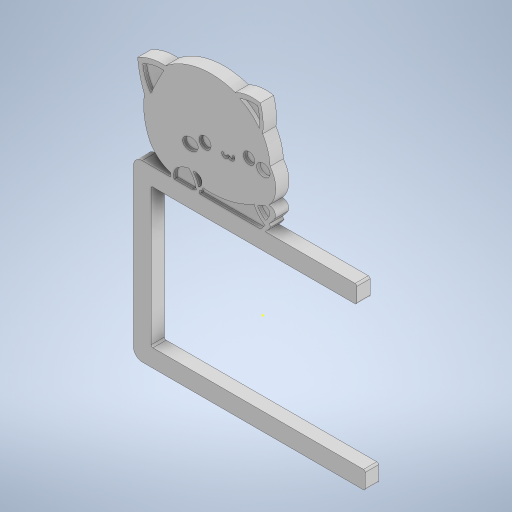
# Autodesk Inventor part: Top_Left
Saved by Autodesk Inventor 2023 (Build 270158000, 158)
## iProperties
Created: 2022-11-13
Part Number: Top_Left
Material: Generic
Document SubType Name: Modeling
Designer: reide
Density: 1 g/cm^3
Appearance: Default
Author: reide
Autodesk Inventor part; units mm, degrees
ref_plane "YZ Plane" through (0, 0, 0) normal (1, 0, 0) x (0, 1, 0)
ref_plane "XZ Plane" through (0, 0, 0) normal (0, 1, 0) x (-1, 0, 0)
ref_plane "XY Plane" through (0, 0, 0) normal (0, 0, 1) x (1, 0, 0)
sketch "Sketch1" plane through (0, 0, 0) normal (0, 0, 1) x (1, 0, 0)
  line L0 (44.2692, 42.6) -> (44.2692, 40.35) projected
  arc A0 (44.2692, 40.35) -> (45.2692, 39.35) centre (45.2692, 40.35) ccw projected
  line L1 (45.2692, 39.35) -> (59.7692, 39.35) projected
  arc A1 (59.7692, 39.35) -> (60.7692, 40.35) centre (59.7692, 40.35) ccw projected
  line L2 (60.7692, 40.35) -> (60.7692, 48.35) projected
  arc A2 (60.7692, 48.35) -> (59.7692, 49.35) centre (59.7692, 48.35) ccw projected
  line L3 (59.7692, 49.35) -> (-60.5312, 49.35) projected
  arc A3 (-60.5312, 49.35) -> (-65.5312, 44.35) centre (-60.5312, 44.35) ccw projected
  line L4 (-65.5312, 44.35) -> (-65.5312, -44.35) projected
  arc A4 (-65.5312, -44.35) -> (-60.5312, -49.35) centre (-60.5312, -44.35) ccw projected
  line L5 (-60.5312, -49.35) -> (64.5312, -49.35) projected
  arc A5 (64.5312, -49.35) -> (65.5312, -48.35) centre (64.5312, -48.35) ccw projected
  line L6 (65.5312, -48.35) -> (65.5312, -40.35) projected
  arc A6 (65.5312, -40.35) -> (64.5312, -39.35) centre (64.5312, -40.35) ccw projected
  line L7 (64.5312, -39.35) -> (49.5062, -39.35) projected
  line L8 (49.5062, -39.35) -> (49.5062, -41.65) projected
  arc A7 (48.5062, -42.65) -> (49.5062, -41.65) centre (48.5062, -41.65) ccw projected
  line L9 (48.5062, -42.65) -> (29.9062, -42.65) projected
  arc A8 (28.9062, -41.65) -> (29.9062, -42.65) centre (29.9062, -41.65) ccw projected
  line L10 (28.9062, -41.65) -> (28.9062, -39.35) projected
  line L11 (28.9062, -39.35) -> (-18.4058, -39.35) projected
  line L12 (-18.4058, -39.35) -> (-18.4058, -41.65) projected
  arc A9 (-19.4058, -42.65) -> (-18.4058, -41.65) centre (-19.4058, -41.65) ccw projected
  line L13 (-19.4058, -42.65) -> (-38.0058, -42.65) projected
  arc A10 (-39.0058, -41.65) -> (-38.0058, -42.65) centre (-38.0058, -41.65) ccw projected
  line L14 (-39.0058, -41.65) -> (-39.0058, -39.35) projected
  line L15 (-39.0058, -39.35) -> (-54.5312, -39.35) projected
  arc A11 (-55.5312, -38.35) -> (-54.5312, -39.35) centre (-54.5312, -38.35) ccw projected
  line L16 (-55.5312, -38.35) -> (-55.5312, -17.1) projected
  arc A12 (-55.5312, -17.1) -> (-56.5312, -16.1) centre (-56.5312, -17.1) ccw projected
  line L17 (-56.5312, -16.1) -> (-58.7812, -16.1) projected
  arc A13 (-59.7812, -15.1) -> (-58.7812, -16.1) centre (-58.7812, -15.1) ccw projected
  line L18 (-59.7812, -15.1) -> (-59.7812, -4.1) projected
  arc A14 (-58.7812, -3.1) -> (-59.7812, -4.1) centre (-58.7812, -4.1) ccw projected
  line L19 (-58.7812, -3.1) -> (-56.5312, -3.1) projected
  arc A15 (-56.5312, -3.1) -> (-55.5312, -2.1) centre (-56.5312, -2.1) ccw projected
  line L20 (-55.5312, -2.1) -> (-55.5312, 2.225) projected
  line L21 (-55.5312, 2.225) -> (-57.8308, 2.225) projected
  arc A16 (-58.8308, 3.225) -> (-57.8308, 2.225) centre (-57.8308, 3.225) ccw projected
  line L22 (-58.8308, 3.225) -> (-58.8308, 21.825) projected
  arc A17 (-57.8308, 22.825) -> (-58.8308, 21.825) centre (-57.8308, 21.825) ccw projected
  line L23 (-57.8308, 22.825) -> (-55.5312, 22.825) projected
  line L24 (-55.5312, 22.825) -> (-55.5312, 38.35) projected
  arc A18 (-54.5312, 39.35) -> (-55.5312, 38.35) centre (-54.5312, 38.35) ccw projected
  line L25 (-54.5312, 39.35) -> (-39.0058, 39.35) projected
  line L26 (-39.0058, 39.35) -> (-39.0058, 41.65) projected
  arc A19 (-38.0058, 42.65) -> (-39.0058, 41.65) centre (-38.0058, 41.65) ccw projected
  line L27 (-38.0058, 42.65) -> (-19.4058, 42.65) projected
  arc A20 (-18.4058, 41.65) -> (-19.4058, 42.65) centre (-19.4058, 41.65) ccw projected
  line L28 (-18.4058, 41.65) -> (-18.4058, 39.35) projected
  line L29 (-18.4058, 39.35) -> (0.3317, 39.35) projected
  line L30 (0.3317, 39.35) -> (0.3317, 41.65) projected
  arc A21 (1.3317, 42.65) -> (0.3317, 41.65) centre (1.3317, 41.65) ccw projected
  line L31 (1.3317, 42.65) -> (19.9317, 42.65) projected
  arc A22 (20.9317, 41.65) -> (19.9317, 42.65) centre (19.9317, 41.65) ccw projected
  line L32 (20.9317, 41.65) -> (20.9317, 39.35) projected
  line L33 (20.9317, 39.35) -> (25.2692, 39.35) projected
  arc A23 (25.2692, 39.35) -> (26.2692, 40.35) centre (25.2692, 40.35) ccw projected
  line L34 (26.2692, 40.35) -> (26.2692, 42.35) projected
  arc A24 (25.2692, 41.35) -> (26.2692, 42.35) centre (25.2692, 42.35) ccw projected
  line L35 (25.2692, 41.35) -> (21.9317, 41.35) projected
  arc A25 (20.9317, 42.35) -> (21.9317, 41.35) centre (21.9317, 42.35) ccw projected
  line L36 (20.9317, 44.2959) -> (20.9317, 42.35) projected
  ellipse E0 centre (21.9317, 44.2959) end of major axis (21.9317, 43.2418) minor radius 1 (21.9317, 45.35) -> (20.9317, 44.2959) ccw projected
  line L37 (21.9317, 45.35) -> (34.9317, 45.35) projected
  ellipse E1 centre (34.9317, 44.2959) end of major axis (34.9317, 43.2418) minor radius 1 (35.9207, 44.452) -> (34.9317, 45.35) ccw projected
  arc A26 (34.9317, 43.6) -> (35.9207, 44.452) centre (34.9317, 44.6) ccw projected
  line L38 (34.9317, 43.6) -> (43.2692, 43.6) projected
  arc A27 (44.2692, 42.6) -> (43.2692, 43.6) centre (43.2692, 42.6) ccw projected
  arc A28 (-39.0058, -42.35) -> (-40.0058, -41.35) centre (-40.0058, -42.35) ccw projected
  line L39 (-39.0058, -44.2959) -> (-39.0058, -42.35) projected
  ellipse E2 centre (-40.0058, -44.2959) end of major axis (-40.0058, -43.2418) minor radius 1 (-40.0058, -45.35) -> (-39.0058, -44.2959) ccw projected
  line L40 (-40.0058, -45.35) -> (-53.0057, -45.35) projected
  ellipse E3 centre (-53.0057, -44.2959) end of major axis (-53.0057, -43.2418) minor radius 1 (-54.0057, -44.2959) -> (-53.0057, -45.35) ccw projected
  line L41 (-54.0057, -42.35) -> (-54.0057, -44.2959) projected
  arc A29 (-53.0057, -41.35) -> (-54.0057, -42.35) centre (-53.0057, -42.35) ccw projected
  line L42 (-53.0057, -41.35) -> (-40.0058, -41.35) projected
  circle A30 centre (55.7692, 44.35) radius 2.125 projected
  circle A31 centre (-60.5312, 44.35) radius 2.125 projected
  circle A32 centre (-60.5312, -44.35) radius 2.125 projected
  circle A33 centre (60.5312, -44.35) radius 2.125 projected
  line L43 (-40.0058, 41.35) -> (-53.0058, 41.35) projected
  arc A34 (-54.0058, 42.35) -> (-53.0058, 41.35) centre (-53.0058, 42.35) ccw projected
  line L44 (-54.0058, 44.2959) -> (-54.0058, 42.35) projected
  ellipse E4 centre (-53.0058, 44.2959) end of major axis (-53.0058, 43.2418) minor radius 1 (-53.0058, 45.35) -> (-54.0058, 44.2959) ccw projected
  line L45 (-53.0058, 45.35) -> (-40.0058, 45.35) projected
  ellipse E5 centre (-40.0058, 44.2959) end of major axis (-40.0058, 43.2418) minor radius 1 (-39.0058, 44.2959) -> (-40.0058, 45.35) ccw projected
  line L46 (-39.0058, 42.35) -> (-39.0058, 44.2959) projected
  arc A35 (-40.0058, 41.35) -> (-39.0058, 42.35) centre (-40.0058, 42.35) ccw projected
  arc A36 (28.9062, -42.35) -> (27.9062, -41.35) centre (27.9062, -42.35) ccw projected
  line L47 (28.9062, -44.2959) -> (28.9062, -42.35) projected
  ellipse E6 centre (27.9062, -44.2959) end of major axis (27.9062, -43.2418) minor radius 1 (27.9063, -45.35) -> (28.9062, -44.2959) ccw projected
  line L48 (27.9063, -45.35) -> (14.9063, -45.35) projected
  ellipse E7 centre (14.9063, -44.2959) end of major axis (14.9063, -43.2418) minor radius 1 (13.9063, -44.2959) -> (14.9063, -45.35) ccw projected
  line L49 (13.9063, -42.35) -> (13.9063, -44.2959) projected
  arc A37 (14.9063, -41.35) -> (13.9063, -42.35) centre (14.9063, -42.35) ccw projected
  line L50 (14.9063, -41.35) -> (27.9062, -41.35) projected
  line L51 (-39.0058, 39.35) -> (45.2692, 39.35)
  line L52 (-55.5312, 22.825) -> (-55.5312, -17.1)
  line L53 (-39.0058, -39.35) -> (49.5062, -39.35)
  point P0 (0, 0)
  point P1 (-55.5312, 2.225)
  constraints: 6 end point, 2 perpendicular, 1 horizontal, 8 other
extrude "Extrusion1" add sketch "Sketch1" along normal blind 7.5 contours A27 L38 A26 E1 L37 E0 L36 A25 L35 A24 L34 A23 L33 L32 A22 L31 A21 L30 L29 L28 A20 L27 A19 L26 L25 A18 L24 L23 A17 L22 A16 L21 L20 A15 L19 A14 L18 A13 L17 A12 L16 A11 L15 L14 A10 L13 A9 L12 L11 L10 A8 L9 A7 L8 L7 A6 L6 A5 L5 A4 L4 A3 L3 A2 L2 A1 L1 A0 L0 | L0 A0 L51 A23 L34 A24 L35 A25 L36 E0 L37 E1 A26 L38 A27 | L51 L30 A21 L31 A22 L32 | L51 L26 A19 L27 A20 L28 | L52 L21 A16 L22 A17 L23 | L52 A12 L17 A13 L18 A14 L19 A15 | L8 A7 L9 A8 L10 L53 | L53 L12 A9 L13 A10 L14 | L39 E2 L40 E3 L41 A29 L42 A28 | A30 | A31 | A32 | A33 | L43 A34 L44 E4 L45 E5 L46 A35 | L47 E6 L48 E7 L49 A37 L50 A36
sketch "Sketch3" plane through (65.5312, -48.35, 0) normal (1, 0, 0) x (0, 0, -1)
  line L0 (0, 9) -> (0, 7)
  line L1 (0, 7) -> (-3, 7)
  line L2 (-3, 7) -> (-3, 1.7)
  line L3 (0, 7) -> (0, 2.7)
  line L4 (0, 2.7) -> (-3, 1.7)
  line L5 (0, 48.35) -> (-9, 48.35)
  line L6 (0, 97.7) -> (-5.5, 97.7)
  line L7 (0, 87.7) -> (-5.5, 87.7)
  line L8 (0, 87.7) -> (0, 89.7)
  line L9 (0, 89.7) -> (-3, 89.7)
  line L10 (-3, 89.7) -> (-3, 95)
  line L11 (0, 89.7) -> (0, 94)
  line L12 (0, 90.575) -> (0, 94.825)
  line L13 (0, 94) -> (-3, 95)
  point P0 (0, -1)
  point P1 (0, 6.125)
  point P2 (0, 1.875)
  dimension "d5" = 2
  dimension "d6" = 3
  dimension "d7" = 5.3
  dimension "d8" = 4.3
  constraints: 28 end point, 8 symmetric about line, 2 vertical, 1 horizontal, 1 perpendicular, 1 point on line
  measures "d5" distance of L0.start L0.end
  measures "d6" distance of L0.end L1.end
  measures "d7" distance of L1.end L2.end
  measures "d8" distance of L0.end L3.end
extrude "Extrusion3" cut sketch "Sketch3" against normal up to surface (131.0625 mm away)
sketch "Sketch4" plane through (0, 0, 0) normal (0, 0, -1) x (-1, 0, 0)
  point P0 (0, 0)
sketch "Sketch5" plane through (0, 0, 0) normal (0, 0, -1) x (-1, 0, 0)
  line L0 (54.0057, -42.35) -> (54.0057, -44.2959) projected
  line L1 (39.0058, -44.2959) -> (39.0058, -42.35) projected
  line L2 (-28.9062, -44.2959) -> (-28.9062, -42.35) projected
  line L3 (-13.9063, -42.35) -> (-13.9063, -44.2959) projected
  line L4 (-44.2692, 42.6) -> (-44.2692, 40.35) projected
  arc A0 (-45.2692, 39.35) -> (-44.2692, 40.35) centre (-45.2692, 40.35) ccw projected
  line L5 (-45.2692, 39.35) -> (-59.7692, 39.35) projected
  arc A1 (-60.7692, 40.35) -> (-59.7692, 39.35) centre (-59.7692, 40.35) ccw projected
  line L6 (-60.7692, 40.35) -> (-60.7692, 48.35) projected
  arc A2 (-59.7692, 49.35) -> (-60.7692, 48.35) centre (-59.7692, 48.35) ccw projected
  line L7 (-59.7692, 49.35) -> (60.5312, 49.35) projected
  arc A3 (65.5312, 44.35) -> (60.5312, 49.35) centre (60.5312, 44.35) ccw projected
  line L8 (65.5312, 44.35) -> (65.5312, -44.35) projected
  arc A4 (60.5312, -49.35) -> (65.5312, -44.35) centre (60.5312, -44.35) ccw projected
  line L9 (60.5312, -49.35) -> (-64.5312, -49.35) projected
  arc A5 (-65.5312, -48.35) -> (-64.5312, -49.35) centre (-64.5312, -48.35) ccw projected
  line L10 (-65.5312, -48.35) -> (-65.5312, -40.35) projected
  arc A6 (-64.5312, -39.35) -> (-65.5312, -40.35) centre (-64.5312, -40.35) ccw projected
  line L11 (-64.5312, -39.35) -> (-49.5062, -39.35) projected
  line L12 (-49.5062, -39.35) -> (-49.5062, -41.65) projected
  arc A7 (-49.5062, -41.65) -> (-48.5062, -42.65) centre (-48.5062, -41.65) ccw projected
  line L13 (-48.5062, -42.65) -> (-29.9062, -42.65) projected
  arc A8 (-29.9062, -42.65) -> (-28.9062, -41.65) centre (-29.9062, -41.65) ccw projected
  line L14 (-28.9062, -41.65) -> (-28.9062, -39.35) projected
  line L15 (-28.9062, -39.35) -> (18.4058, -39.35) projected
  line L16 (18.4058, -39.35) -> (18.4058, -41.65) projected
  arc A9 (18.4058, -41.65) -> (19.4058, -42.65) centre (19.4058, -41.65) ccw projected
  line L17 (19.4058, -42.65) -> (38.0058, -42.65) projected
  arc A10 (38.0058, -42.65) -> (39.0058, -41.65) centre (38.0058, -41.65) ccw projected
  line L18 (39.0058, -41.65) -> (39.0058, -39.35) projected
  line L19 (39.0058, -39.35) -> (54.5312, -39.35) projected
  arc A11 (54.5312, -39.35) -> (55.5312, -38.35) centre (54.5312, -38.35) ccw projected
  line L20 (55.5312, -38.35) -> (55.5312, -17.1) projected
  arc A12 (56.5312, -16.1) -> (55.5312, -17.1) centre (56.5312, -17.1) ccw projected
  line L21 (56.5312, -16.1) -> (58.7812, -16.1) projected
  arc A13 (58.7812, -16.1) -> (59.7812, -15.1) centre (58.7812, -15.1) ccw projected
  line L22 (59.7812, -15.1) -> (59.7812, -4.1) projected
  arc A14 (59.7812, -4.1) -> (58.7812, -3.1) centre (58.7812, -4.1) ccw projected
  line L23 (58.7812, -3.1) -> (56.5312, -3.1) projected
  arc A15 (55.5312, -2.1) -> (56.5312, -3.1) centre (56.5312, -2.1) ccw projected
  line L24 (55.5312, -2.1) -> (55.5312, 2.225) projected
  line L25 (55.5312, 2.225) -> (57.8308, 2.225) projected
  arc A16 (57.8308, 2.225) -> (58.8308, 3.225) centre (57.8308, 3.225) ccw projected
  line L26 (58.8308, 3.225) -> (58.8308, 21.825) projected
  arc A17 (58.8308, 21.825) -> (57.8308, 22.825) centre (57.8308, 21.825) ccw projected
  line L27 (57.8308, 22.825) -> (55.5312, 22.825) projected
  line L28 (55.5312, 22.825) -> (55.5312, 38.35) projected
  arc A18 (55.5312, 38.35) -> (54.5312, 39.35) centre (54.5312, 38.35) ccw projected
  line L29 (54.5312, 39.35) -> (39.0058, 39.35) projected
  line L30 (39.0058, 39.35) -> (39.0058, 41.65) projected
  arc A19 (39.0058, 41.65) -> (38.0058, 42.65) centre (38.0058, 41.65) ccw projected
  line L31 (38.0058, 42.65) -> (19.4058, 42.65) projected
  arc A20 (19.4058, 42.65) -> (18.4058, 41.65) centre (19.4058, 41.65) ccw projected
  line L32 (18.4058, 41.65) -> (18.4058, 39.35) projected
  line L33 (18.4058, 39.35) -> (-0.3317, 39.35) projected
  line L34 (-0.3317, 39.35) -> (-0.3317, 41.65) projected
  arc A21 (-0.3317, 41.65) -> (-1.3317, 42.65) centre (-1.3317, 41.65) ccw projected
  line L35 (-1.3317, 42.65) -> (-19.9317, 42.65) projected
  arc A22 (-19.9317, 42.65) -> (-20.9317, 41.65) centre (-19.9317, 41.65) ccw projected
  line L36 (-20.9317, 41.65) -> (-20.9317, 39.35) projected
  line L37 (-20.9317, 39.35) -> (-25.2692, 39.35) projected
  arc A23 (-26.2692, 40.35) -> (-25.2692, 39.35) centre (-25.2692, 40.35) ccw projected
  line L38 (-26.2692, 40.35) -> (-26.2692, 42.35) projected
  arc A24 (-26.2692, 42.35) -> (-25.2692, 41.35) centre (-25.2692, 42.35) ccw projected
  line L39 (-25.2692, 41.35) -> (-21.9317, 41.35) projected
  arc A25 (-21.9317, 41.35) -> (-20.9317, 42.35) centre (-21.9317, 42.35) ccw projected
  line L40 (-20.9317, 44.2959) -> (-20.9317, 42.35) projected
  ellipse E0 centre (-21.9317, 44.2959) end of major axis (-21.9317, 43.2418) minor radius 1 (-20.9317, 44.2959) -> (-21.9317, 45.35) ccw projected
  line L41 (-21.9317, 45.35) -> (-34.9317, 45.35) projected
  ellipse E1 centre (-34.9317, 44.2959) end of major axis (-34.9317, 43.2418) minor radius 1 (-34.9317, 45.35) -> (-35.9207, 44.452) ccw projected
  arc A26 (-35.9207, 44.452) -> (-34.9317, 43.6) centre (-34.9317, 44.6) ccw projected
  line L42 (-34.9317, 43.6) -> (-43.2692, 43.6) projected
  arc A27 (-43.2692, 43.6) -> (-44.2692, 42.6) centre (-43.2692, 42.6) ccw projected
  arc A28 (40.0058, -41.35) -> (39.0058, -42.35) centre (40.0058, -42.35) ccw projected
  line L43 (39.0058, -44.2959) -> (39.0058, -42.35) projected
  ellipse E2 centre (40.0058, -44.2959) end of major axis (40.0058, -43.2418) minor radius 1 (39.0058, -44.2959) -> (40.0058, -45.35) ccw projected
  line L44 (40.0058, -45.35) -> (53.0057, -45.35) projected
  ellipse E3 centre (53.0057, -44.2959) end of major axis (53.0057, -43.2418) minor radius 1 (53.0057, -45.35) -> (54.0057, -44.2959) ccw projected
  line L45 (54.0057, -42.35) -> (54.0057, -44.2959) projected
  arc A29 (54.0057, -42.35) -> (53.0057, -41.35) centre (53.0057, -42.35) ccw projected
  line L46 (53.0057, -41.35) -> (40.0058, -41.35) projected
  circle A30 centre (-55.7692, 44.35) radius 2.125 projected
  circle A31 centre (60.5312, 44.35) radius 2.125 projected
  circle A32 centre (60.5312, -44.35) radius 2.125 projected
  circle A33 centre (-60.5312, -44.35) radius 2.125 projected
  line L47 (40.0058, 41.35) -> (53.0058, 41.35) projected
  arc A34 (53.0058, 41.35) -> (54.0058, 42.35) centre (53.0058, 42.35) ccw projected
  line L48 (54.0058, 44.2959) -> (54.0058, 42.35) projected
  ellipse E4 centre (53.0058, 44.2959) end of major axis (53.0058, 43.2418) minor radius 1 (54.0058, 44.2959) -> (53.0058, 45.35) ccw projected
  line L49 (53.0058, 45.35) -> (40.0058, 45.35) projected
  ellipse E5 centre (40.0058, 44.2959) end of major axis (40.0058, 43.2418) minor radius 1 (40.0058, 45.35) -> (39.0058, 44.2959) ccw projected
  line L50 (39.0058, 42.35) -> (39.0058, 44.2959) projected
  arc A35 (39.0058, 42.35) -> (40.0058, 41.35) centre (40.0058, 42.35) ccw projected
  arc A36 (-27.9062, -41.35) -> (-28.9062, -42.35) centre (-27.9062, -42.35) ccw projected
  line L51 (-28.9062, -44.2959) -> (-28.9062, -42.35) projected
  ellipse E6 centre (-27.9062, -44.2959) end of major axis (-27.9062, -43.2418) minor radius 1 (-28.9062, -44.2959) -> (-27.9063, -45.35) ccw projected
  line L52 (-27.9063, -45.35) -> (-14.9063, -45.35) projected
  ellipse E7 centre (-14.9063, -44.2959) end of major axis (-14.9063, -43.2418) minor radius 1 (-14.9063, -45.35) -> (-13.9063, -44.2959) ccw projected
  line L53 (-13.9063, -42.35) -> (-13.9063, -44.2959) projected
  arc A37 (-13.9063, -42.35) -> (-14.9063, -41.35) centre (-14.9063, -42.35) ccw projected
  line L54 (-14.9063, -41.35) -> (-27.9062, -41.35) projected
  arc A38 (64.9708, -46.65) -> (65.5312, -44.35) centre (60.5312, -44.35) ccw projected
  line L55 (65.5312, -41.35) -> (65.5312, -44.35) projected
  line L56 (-65.5312, -41.35) -> (65.5312, -41.35) projected
  line L57 (-65.5312, -46.65) -> (-65.5312, -41.35) projected
  line L58 (-65.5312, -46.65) -> (64.9708, -46.65) projected
  line L59 (54.0058, -46.65) -> (39.0058, -46.65)
  line L60 (39.0058, -46.65) -> (39.0058, -41.35)
  line L61 (39.0058, -41.35) -> (54.0058, -41.35)
  line L62 (54.0058, -41.35) -> (54.0058, -46.65)
  line L63 (39.0058, -46.65) -> (23.0058, -46.65)
  line L64 (23.0058, -46.65) -> (23.0058, -41.35)
  line L65 (23.0058, -41.35) -> (39.0058, -41.35)
  line L66 (39.0058, -41.35) -> (39.0058, -46.65)
  line L67 (-13.9063, -41.35) -> (-28.9062, -41.35)
  line L68 (-28.9062, -41.35) -> (-28.9063, -46.65)
  line L69 (-28.9063, -46.65) -> (-13.9063, -46.65)
  line L70 (-13.9063, -46.65) -> (-13.9063, -41.35)
  line L71 (-28.9062, -41.35) -> (-44.9063, -41.35)
  line L72 (-44.9063, -41.35) -> (-44.9063, -46.65)
  line L73 (-44.9063, -46.65) -> (-28.9063, -46.65)
  line L74 (-28.9063, -46.65) -> (-28.9062, -41.35)
  line L75 (-60.7692, 46.65) -> (64.9708, 46.65) projected
  line L76 (65.5312, 41.35) -> (-60.7692, 41.35) projected
  line L77 (-60.7692, 41.35) -> (65.5312, 41.35) projected
  line L78 (54.0058, 41.35) -> (39.0058, 41.35)
  line L79 (39.0058, 41.35) -> (39.0058, 46.65)
  line L80 (39.0058, 46.65) -> (54.0058, 46.65)
  line L81 (54.0058, 46.65) -> (54.0058, 41.35)
  line L82 (39.0058, 46.65) -> (23.0058, 46.65)
  line L83 (23.0058, 46.65) -> (23.0058, 41.35)
  line L84 (23.0058, 41.35) -> (39.0058, 41.35)
  line L85 (39.0058, 41.35) -> (39.0058, 46.65)
  line L86 (-20.9317, 41.35) -> (-35.9317, 41.35)
  line L87 (-35.9317, 41.35) -> (-35.9317, 46.65)
  line L88 (-35.9317, 46.65) -> (-20.9317, 46.65)
  line L89 (-20.9317, 46.65) -> (-20.9317, 41.35)
  line L90 (-35.9317, 41.35) -> (-51.9317, 41.35)
  line L91 (-51.9317, 41.35) -> (-51.9317, 46.65)
  line L92 (-51.9317, 46.65) -> (-35.9317, 46.65)
  line L93 (-35.9317, 46.65) -> (-35.9317, 41.35)
  point P0 (0, 0)
  point P1 (23.0058, 46.65)
  point P2 (-20.9317, 46.65)
  point P3 (54.0058, 46.65)
  point P4 (-65.5312, -46.65)
  point P5 (-13.9063, -46.65)
  point P6 (23.0058, -46.65)
  point P7 (64.9708, -46.65)
  dimension "d11" = 16
  dimension "d12" = 15
  dimension "d13" = 16
  dimension "d14" = 15
  dimension "d15" = 16
  constraints: 64 end point, 16 parallel, 13 point on line, 8 horizontal, 8 perpendicular, 8 other
  measures "d11" distance between parallel lines of L64 L66
  measures "d12" distance between parallel lines of L74 L70
  measures "d13" distance between parallel lines of L72 L68
  measures "d14" distance between parallel lines of L87 L89
  measures "d15" distance between parallel lines of L91 L93
extrude "Extrusion4" add sketch "Sketch5" against normal up to surface (3 mm away) contours L62 L56 L8 A4 L58 L0 | L76 L81 L48 L75 A3 L8 | L58 L70 L3 L56 L16 A9 L17 L64 | L64 L17 A9 L16 L56 | L58 L10 L56 L12 A7 L13 L72 | L13 A7 L12 L56 L72 | L83 L31 A20 L32 L76 L34 A21 L35 A22 L89 L40 L75 | L76 L32 A20 L31 L83 | L75 L91 L76 L6 | L76 L36 A22 L35 A21 L34 | A30 | A31 | A32 | A33
sketch "Sketch6" plane through (0, 0, 0) normal (0, 0, -1) x (-1, 0, 0)
  line L0 (-65.5312, -48.35) -> (-65.5312, -40.35) projected
  arc A0 (-65.5312, -48.35) -> (-64.5312, -49.35) centre (-64.5312, -48.35) ccw projected
  line L1 (60.5312, -49.35) -> (-64.5312, -49.35) projected
  arc A1 (60.5312, -49.35) -> (65.5312, -44.35) centre (60.5312, -44.35) ccw projected
  arc A2 (65.5312, 44.35) -> (60.5312, 49.35) centre (60.5312, 44.35) ccw projected
  line L2 (-59.7692, 49.35) -> (60.5312, 49.35) projected
  arc A3 (-59.7692, 49.35) -> (-60.7692, 48.35) centre (-59.7692, 48.35) ccw projected
  line L3 (-60.7692, 40.35) -> (-60.7692, 48.35) projected
  arc A4 (-60.7692, 40.35) -> (-59.7692, 39.35) centre (-59.7692, 40.35) ccw projected
  line L4 (54.5312, 39.35) -> (-59.7692, 39.35) projected
  arc A5 (55.5312, 38.35) -> (54.5312, 39.35) centre (54.5312, 38.35) ccw projected
  line L5 (55.5312, -38.35) -> (55.5312, 38.35) projected
  arc A6 (54.5312, -39.35) -> (55.5312, -38.35) centre (54.5312, -38.35) ccw projected
  line L6 (-64.5312, -39.35) -> (54.5312, -39.35) projected
  arc A7 (-64.5312, -39.35) -> (-65.5312, -40.35) centre (-64.5312, -40.35) ccw projected
  line L7 (-44.9063, -45.65) -> (-44.9063, -41.35) projected
  line L8 (-44.9063, -41.35) -> (-13.9063, -41.35) projected
  line L9 (-13.9063, -41.35) -> (-13.9063, -45.65) projected
  line L10 (-13.9063, -45.65) -> (-44.9063, -45.65) projected
  line L11 (-20.9317, 41.35) -> (-51.9317, 41.35) projected
  line L12 (-51.9317, 41.35) -> (-51.9317, 45.65) projected
  line L13 (-51.9317, 45.65) -> (-20.9317, 45.65) projected
  line L14 (-20.9317, 45.65) -> (-20.9317, 41.35) projected
  line L15 (54.0058, -41.35) -> (54.0058, -45.65) projected
  line L16 (54.0058, -45.65) -> (23.0058, -45.65) projected
  line L17 (23.0058, -45.65) -> (23.0058, -41.35) projected
  line L18 (23.0058, -41.35) -> (54.0058, -41.35) projected
  line L19 (23.0058, 41.35) -> (23.0058, 45.65) projected
  line L20 (23.0058, 45.65) -> (54.0058, 45.65) projected
  line L21 (54.0058, 45.65) -> (54.0058, 41.35) projected
  line L22 (54.0058, 41.35) -> (23.0058, 41.35) projected
  line L23 (-44.2692, 42.6) -> (-44.2692, 40.35) projected
  arc A8 (-45.2692, 39.35) -> (-44.2692, 40.35) centre (-45.2692, 40.35) ccw projected
  line L24 (-45.2692, 39.35) -> (-59.7692, 39.35) projected
  arc A9 (-60.7692, 40.35) -> (-59.7692, 39.35) centre (-59.7692, 40.35) ccw projected
  line L25 (-60.7692, 40.35) -> (-60.7692, 48.35) projected
  arc A10 (-59.7692, 49.35) -> (-60.7692, 48.35) centre (-59.7692, 48.35) ccw projected
  line L26 (-59.7692, 49.35) -> (60.5312, 49.35) projected
  arc A11 (65.5312, 44.35) -> (60.5312, 49.35) centre (60.5312, 44.35) ccw projected
  line L27 (65.5312, 44.35) -> (65.5312, -44.35) projected
  arc A12 (60.5312, -49.35) -> (65.5312, -44.35) centre (60.5312, -44.35) ccw projected
  line L28 (60.5312, -49.35) -> (-64.5312, -49.35) projected
  arc A13 (-65.5312, -48.35) -> (-64.5312, -49.35) centre (-64.5312, -48.35) ccw projected
  line L29 (-65.5312, -48.35) -> (-65.5312, -40.35) projected
  arc A14 (-64.5312, -39.35) -> (-65.5312, -40.35) centre (-64.5312, -40.35) ccw projected
  line L30 (-64.5312, -39.35) -> (-49.5062, -39.35) projected
  line L31 (-49.5062, -39.35) -> (-49.5062, -41.65) projected
  arc A15 (-49.5062, -41.65) -> (-48.5062, -42.65) centre (-48.5062, -41.65) ccw projected
  line L32 (-48.5062, -42.65) -> (-29.9062, -42.65) projected
  arc A16 (-29.9062, -42.65) -> (-28.9062, -41.65) centre (-29.9062, -41.65) ccw projected
  line L33 (-28.9062, -41.65) -> (-28.9062, -39.35) projected
  line L34 (-28.9062, -39.35) -> (18.4058, -39.35) projected
  line L35 (18.4058, -39.35) -> (18.4058, -41.65) projected
  arc A17 (18.4058, -41.65) -> (19.4058, -42.65) centre (19.4058, -41.65) ccw projected
  line L36 (19.4058, -42.65) -> (38.0058, -42.65) projected
  arc A18 (38.0058, -42.65) -> (39.0058, -41.65) centre (38.0058, -41.65) ccw projected
  line L37 (39.0058, -41.65) -> (39.0058, -39.35) projected
  line L38 (39.0058, -39.35) -> (54.5312, -39.35) projected
  arc A19 (54.5312, -39.35) -> (55.5312, -38.35) centre (54.5312, -38.35) ccw projected
  line L39 (55.5312, -38.35) -> (55.5312, -17.1) projected
  arc A20 (56.5312, -16.1) -> (55.5312, -17.1) centre (56.5312, -17.1) ccw projected
  line L40 (56.5312, -16.1) -> (58.7812, -16.1) projected
  arc A21 (58.7812, -16.1) -> (59.7812, -15.1) centre (58.7812, -15.1) ccw projected
  line L41 (59.7812, -15.1) -> (59.7812, -4.1) projected
  arc A22 (59.7812, -4.1) -> (58.7812, -3.1) centre (58.7812, -4.1) ccw projected
  line L42 (58.7812, -3.1) -> (56.5312, -3.1) projected
  arc A23 (55.5312, -2.1) -> (56.5312, -3.1) centre (56.5312, -2.1) ccw projected
  line L43 (55.5312, -2.1) -> (55.5312, 2.225) projected
  line L44 (55.5312, 2.225) -> (57.8308, 2.225) projected
  arc A24 (57.8308, 2.225) -> (58.8308, 3.225) centre (57.8308, 3.225) ccw projected
  line L45 (58.8308, 3.225) -> (58.8308, 21.825) projected
  arc A25 (58.8308, 21.825) -> (57.8308, 22.825) centre (57.8308, 21.825) ccw projected
  line L46 (57.8308, 22.825) -> (55.5312, 22.825) projected
  line L47 (55.5312, 22.825) -> (55.5312, 38.35) projected
  arc A26 (55.5312, 38.35) -> (54.5312, 39.35) centre (54.5312, 38.35) ccw projected
  line L48 (54.5312, 39.35) -> (39.0058, 39.35) projected
  line L49 (39.0058, 39.35) -> (39.0058, 41.65) projected
  arc A27 (39.0058, 41.65) -> (38.0058, 42.65) centre (38.0058, 41.65) ccw projected
  line L50 (38.0058, 42.65) -> (19.4058, 42.65) projected
  arc A28 (19.4058, 42.65) -> (18.4058, 41.65) centre (19.4058, 41.65) ccw projected
  line L51 (18.4058, 41.65) -> (18.4058, 39.35) projected
  line L52 (18.4058, 39.35) -> (-0.3317, 39.35) projected
  line L53 (-0.3317, 39.35) -> (-0.3317, 41.65) projected
  arc A29 (-0.3317, 41.65) -> (-1.3317, 42.65) centre (-1.3317, 41.65) ccw projected
  line L54 (-1.3317, 42.65) -> (-19.9317, 42.65) projected
  arc A30 (-19.9317, 42.65) -> (-20.9317, 41.65) centre (-19.9317, 41.65) ccw projected
  line L55 (-20.9317, 41.65) -> (-20.9317, 39.35) projected
  line L56 (-20.9317, 39.35) -> (-25.2692, 39.35) projected
  arc A31 (-26.2692, 40.35) -> (-25.2692, 39.35) centre (-25.2692, 40.35) ccw projected
  line L57 (-26.2692, 40.35) -> (-26.2692, 42.35) projected
  arc A32 (-26.2692, 42.35) -> (-25.2692, 41.35) centre (-25.2692, 42.35) ccw projected
  line L58 (-25.2692, 41.35) -> (-21.9317, 41.35) projected
  arc A33 (-21.9317, 41.35) -> (-20.9317, 42.35) centre (-21.9317, 42.35) ccw projected
  line L59 (-20.9317, 44.2959) -> (-20.9317, 42.35) projected
  ellipse E0 centre (-21.9317, 44.2959) end of major axis (-21.9317, 43.2418) minor radius 1 (-20.9317, 44.2959) -> (-21.9317, 45.35) ccw projected
  line L60 (-21.9317, 45.35) -> (-34.9317, 45.35) projected
  ellipse E1 centre (-34.9317, 44.2959) end of major axis (-34.9317, 43.2418) minor radius 1 (-34.9317, 45.35) -> (-35.9207, 44.452) ccw projected
  arc A34 (-35.9207, 44.452) -> (-34.9317, 43.6) centre (-34.9317, 44.6) ccw projected
  line L61 (-34.9317, 43.6) -> (-43.2692, 43.6) projected
  arc A35 (-43.2692, 43.6) -> (-44.2692, 42.6) centre (-43.2692, 42.6) ccw projected
  arc A36 (40.0058, -41.35) -> (39.0058, -42.35) centre (40.0058, -42.35) ccw projected
  line L62 (39.0058, -44.2959) -> (39.0058, -42.35) projected
  ellipse E2 centre (40.0058, -44.2959) end of major axis (40.0058, -43.2418) minor radius 1 (39.0058, -44.2959) -> (40.0058, -45.35) ccw projected
  line L63 (40.0058, -45.35) -> (53.0057, -45.35) projected
  ellipse E3 centre (53.0057, -44.2959) end of major axis (53.0057, -43.2418) minor radius 1 (53.0057, -45.35) -> (54.0057, -44.2959) ccw projected
  line L64 (54.0057, -42.35) -> (54.0057, -44.2959) projected
  arc A37 (54.0057, -42.35) -> (53.0057, -41.35) centre (53.0057, -42.35) ccw projected
  line L65 (53.0057, -41.35) -> (40.0058, -41.35) projected
  circle A38 centre (-55.7692, 44.35) radius 2.125 projected
  circle A39 centre (60.5312, 44.35) radius 2.125 projected
  circle A40 centre (60.5312, -44.35) radius 2.125 projected
  circle A41 centre (-60.5312, -44.35) radius 2.125 projected
  line L66 (40.0058, 41.35) -> (53.0058, 41.35) projected
  arc A42 (53.0058, 41.35) -> (54.0058, 42.35) centre (53.0058, 42.35) ccw projected
  line L67 (54.0058, 44.2959) -> (54.0058, 42.35) projected
  ellipse E4 centre (53.0058, 44.2959) end of major axis (53.0058, 43.2418) minor radius 1 (54.0058, 44.2959) -> (53.0058, 45.35) ccw projected
  line L68 (53.0058, 45.35) -> (40.0058, 45.35) projected
  ellipse E5 centre (40.0058, 44.2959) end of major axis (40.0058, 43.2418) minor radius 1 (40.0058, 45.35) -> (39.0058, 44.2959) ccw projected
  line L69 (39.0058, 42.35) -> (39.0058, 44.2959) projected
  arc A43 (39.0058, 42.35) -> (40.0058, 41.35) centre (40.0058, 42.35) ccw projected
  arc A44 (-27.9062, -41.35) -> (-28.9062, -42.35) centre (-27.9062, -42.35) ccw projected
  line L70 (-28.9062, -44.2959) -> (-28.9062, -42.35) projected
  ellipse E6 centre (-27.9062, -44.2959) end of major axis (-27.9062, -43.2418) minor radius 1 (-28.9062, -44.2959) -> (-27.9063, -45.35) ccw projected
  line L71 (-27.9063, -45.35) -> (-14.9063, -45.35) projected
  ellipse E7 centre (-14.9063, -44.2959) end of major axis (-14.9063, -43.2418) minor radius 1 (-14.9063, -45.35) -> (-13.9063, -44.2959) ccw projected
  line L72 (-13.9063, -42.35) -> (-13.9063, -44.2959) projected
  arc A45 (-13.9063, -42.35) -> (-14.9063, -41.35) centre (-14.9063, -42.35) ccw projected
  line L73 (-14.9063, -41.35) -> (-27.9062, -41.35) projected
  line L74 (39.0058, 41.35) -> (23.0058, 41.35)
  line L75 (23.0058, 41.35) -> (23.0058, 45.65)
  line L76 (23.0058, 45.65) -> (39.0058, 45.65)
  line L77 (39.0058, 45.65) -> (39.0058, 41.35)
  line L78 (-51.9317, 41.35) -> (-35.9317, 41.35)
  line L79 (-35.9317, 41.35) -> (-35.9317, 45.65)
  line L80 (-35.9317, 45.65) -> (-51.9317, 45.65)
  line L81 (-51.9317, 45.65) -> (-51.9317, 41.35)
  line L82 (23.0058, -41.35) -> (54.0058, -41.35) projected
  line L83 (39.0058, -41.35) -> (23.0058, -41.35)
  line L84 (23.0058, -41.35) -> (23.0058, -45.65)
  line L85 (23.0058, -45.65) -> (39.0058, -45.65)
  line L86 (39.0058, -45.65) -> (39.0058, -41.35)
  line L87 (-28.9062, -41.35) -> (-44.9063, -41.35)
  line L88 (-44.9063, -41.35) -> (-44.9063, -45.65)
  line L89 (-44.9063, -45.65) -> (-28.9062, -45.65)
  line L90 (-28.9062, -45.65) -> (-28.9062, -41.35)
  line L91 (-20.9317, 41.35) -> (-20.9317, 46.65) projected
  line L92 (-51.9317, 46.65) -> (-20.9317, 46.65) projected
  line L93 (-51.9317, 46.65) -> (-51.9317, 41.35) projected
  line L94 (-51.9317, 41.35) -> (-20.9317, 41.35) projected
  line L95 (23.0058, 46.65) -> (23.0058, 41.35) projected
  line L96 (23.0058, 41.35) -> (54.0058, 41.35) projected
  line L97 (54.0058, 41.35) -> (54.0058, 46.65) projected
  line L98 (23.0058, 46.65) -> (54.0058, 46.65) projected
  line L99 (-44.9063, -41.35) -> (-44.9063, -46.65) projected
  line L100 (-44.9063, -46.65) -> (-13.9063, -46.65) projected
  line L101 (-13.9063, -46.65) -> (-13.9063, -41.35) projected
  line L102 (-44.9063, -41.35) -> (-13.9063, -41.35) projected
  line L103 (54.0058, -46.65) -> (54.0058, -41.35) projected
  line L104 (23.0058, -41.35) -> (54.0058, -41.35) projected
  line L105 (23.0058, -41.35) -> (23.0058, -46.65) projected
  line L106 (23.0058, -46.65) -> (54.0058, -46.65) projected
  line L107 (39.0058, -46.65) -> (23.0058, -46.65)
  line L108 (23.0058, -46.65) -> (23.0058, -41.35)
  line L109 (23.0058, -41.35) -> (39.0058, -41.35)
  line L110 (39.0058, -41.35) -> (39.0058, -46.65)
  line L111 (-28.9062, -46.65) -> (-44.9063, -46.65)
  line L112 (-44.9063, -46.65) -> (-44.9063, -41.35)
  line L113 (-44.9063, -41.35) -> (-28.9062, -41.35)
  line L114 (-28.9062, -41.35) -> (-28.9062, -46.65)
  line L115 (-35.9317, 41.35) -> (-51.9317, 41.35)
  line L116 (-51.9317, 41.35) -> (-51.9317, 46.65)
  line L117 (-51.9317, 46.65) -> (-35.9317, 46.65)
  line L118 (-35.9317, 46.65) -> (-35.9317, 41.35)
  line L119 (39.0058, 41.35) -> (23.0058, 41.35)
  line L120 (23.0058, 41.35) -> (23.0058, 46.65)
  line L121 (23.0058, 46.65) -> (39.0058, 46.65)
  line L122 (39.0058, 46.65) -> (39.0058, 41.35)
  line L123 (65.5312, 44.35) -> (65.5312, -44.35) projected
  point P0 (0, 0)
  point P1 (39.0058, 46.65)
  point P2 (-35.9317, 46.65)
  point P3 (-28.9062, -45.65)
  point P4 (-28.9062, -42.35)
  dimension "d18" = 16
  constraints: 64 end point, 16 parallel, 9 point on line, 8 horizontal, 8 perpendicular, 8 other
  measures "d18" distance between parallel lines of L12 L79
extrude "Extrusion5" cut sketch "Sketch6" against normal up to surface (3 mm away) contours L33 A16 L32 L7 L8 | L90 L70 L10 L7 L32 A16 | L37 A18 L36 L17 L18 | L10 L114 L100 L99 | L86 L62 L16 L17 L36 A18 | L16 L110 L106 L105 | L23 A35 L61 L79 L11 | L11 L12 L13 L79 L61 A35 L23 | L93 L92 L118 L13 | L22 L19 L50 A27 L49 | A27 L50 L19 L20 L77 L69 | L95 L98 L122 L20
sketch "Sketch7" plane through (0, 0, 0) normal (0, 0, -1) x (-1, 0, 0)
  circle A0 centre (60.5312, -44.35) radius 2.125 projected
  circle A1 centre (-60.5312, -44.35) radius 2.125 projected
  circle A2 centre (-55.7692, 44.35) radius 2.125 projected
  circle A3 centre (60.5312, 44.35) radius 2.125 projected
  point P0 (0, 0)
extrude "Extrusion6" cut sketch "Sketch7" against normal blind 1.8
sketch "Sketch8" plane through (0, 0, 7.5) normal (0, 0, 1) x (1, 0, 0)
  line L0 (-67.6586, 125.6846) -> (22.3414, 125.6846) construction
  line L1 (22.3414, 125.6846) -> (22.3414, 35.6846) construction
  line L2 (22.3414, 35.6846) -> (-67.6586, 35.6846) construction
  line L3 (-67.6586, 35.6846) -> (-67.6586, 125.6846) construction
  arc A0 (-41.2311, 56.4471) -> (-43.7668, 46.9111) centre (-36.8862, 50.1866) ccw
  arc A1 (-34.4764, 59.5735) -> (-41.2311, 56.4471) centre (-26.9493, 34.4515) ccw
  arc A2 (-56.18, 60.807) -> (-44.4039, 51.4337) centre (-38.8296, 70.521) ccw
  arc A3 (-59.3268, 82.3482) -> (-56.18, 60.807) centre (-22.274, 76.7606) ccw
  arc A4 (-63.1417, 98.5922) -> (-59.3268, 82.3482) centre (-7.2967, 103.1374) ccw
  arc A5 (-47.4515, 102.3148) -> (-63.1417, 98.5922) centre (-49.1128, 74.3896) ccw
  arc A6 (-7.9799, 108.9908) -> (-47.4515, 102.3148) centre (-21.6467, 69.7703) ccw
  arc A7 (6.1831, 110.8888) -> (-7.9799, 108.9908) centre (1.8063, 89.7576) ccw
  arc A8 (7.5139, 96.445) -> (6.1831, 110.8888) centre (-24.9939, 100.7331) ccw
  arc A9 (11.701, 82.5854) -> (7.5139, 96.445) centre (-17.5403, 81.3137) ccw
  arc A10 (14.3248, 58.2512) -> (9.8656, 63.0979) centre (11.2567, 59.9031) ccw
  arc A11 (11.1906, 63.387) -> (11.701, 82.5854) centre (-0.1255, 73.2938) ccw
  line L4 (67.875, 49.3124) -> (-69.3262, 49.3124)
  arc A12 (-29.0116, 49.3124) -> (-34.4764, 59.5735) centre (-43.5467, 48.1571) ccw
  arc A13 (-29.2093, 50.811) -> (-33.4806, 58.7059) centre (-31.0856, 54.8987) ccw
  arc A14 (12.1204, 53.0639) -> (4.599, 61.1063) centre (-35.0005, 16.5336) ccw
  arc A15 (9.8656, 63.0979) -> (5.7487, 60.0577) centre (20.7308, 44.0772) ccw
  arc A16 (11.1906, 54.2327) -> (14.3248, 58.2512) centre (-10.3438, 74.2601) ccw
  arc A17 (9.0437, 49.3124) -> (12.1204, 53.0639) centre (-3.3832, 62.6419) ccw
  arc A18 (-27.1296, 52.7585) -> (4.599, 61.1063) centre (-24.0439, 105.5019) ccw
  line L5 (59.7692, 49.35) -> (-60.5312, 49.35) projected
  point P0 (0, 0)
  point P1 (-44.4606, 49.35)
  point P2 (9.0839, 49.35)
  dimension "d23" = 90
  constraints: 46 point on circle, 19 centre point, 2 end point, 2 point on line, 1 other
  measures "d23" distance of L2.end L0.start
extrude "Extrusion7" add sketch "Sketch8" against normal up to surface (7.5 mm away) contours A1 A12 L5 A0 | A0 A2 A3 A4 A5 A6 A7 A8 A9 A11 A10 A15 A14 A18 A13 A12 A1 | A13 A12 | A12 A13 A18 A14 A17 L5 | A15 A10 A16 A14
sketch "Sketch9" plane through (0, 0, 7.5) normal (0, 0, 1) x (1, 0, 0)
  line L0 (-67.4615, 125.7619) -> (22.5385, 125.7619) construction
  line L1 (22.5385, 125.7619) -> (22.5385, 35.7619) construction
  line L2 (22.5385, 35.7619) -> (-67.4615, 35.7619) construction
  line L3 (-67.4615, 35.7619) -> (-67.4615, 125.7619) construction
  line L4 (-64.9012, -54.686) -> (-64.9012, 38.3124)
  arc A0 (-63.9012, 39.3124) -> (-64.9012, 38.3124) centre (-63.9012, 38.3124) ccw
  line L5 (-63.9012, 39.3124) -> (67.875, 39.3124)
  arc A1 (67.875, 39.3124) -> (68.875, 40.3124) centre (67.875, 40.3124) ccw
  line L6 (68.875, 40.3124) -> (68.875, 48.3124)
  arc A2 (68.875, 48.3124) -> (67.875, 49.3124) centre (67.875, 48.3124) ccw
  line L7 (67.875, 49.3124) -> (9.0437, 49.3124)
  arc A3 (9.0437, 49.3124) -> (12.1204, 53.0639) centre (-3.3832, 62.6419) ccw
  arc A4 (12.1204, 53.0639) -> (11.1906, 54.2327) centre (-35.0005, 16.5336) ccw
  arc A5 (11.1906, 54.2327) -> (14.3248, 58.2512) centre (-10.3438, 74.2601) ccw
  arc A6 (14.3248, 58.2512) -> (11.1906, 63.387) centre (11.2567, 59.9031) ccw
  arc A7 (11.1906, 63.387) -> (11.701, 82.5854) centre (-0.1255, 73.2938) ccw
  arc A8 (11.701, 82.5854) -> (7.5139, 96.445) centre (-17.5403, 81.3137) ccw
  arc A9 (7.5139, 96.445) -> (6.1831, 110.8888) centre (-24.9939, 100.7331) ccw
  arc A10 (6.1831, 110.8888) -> (-7.9799, 108.9908) centre (1.8063, 89.7576) ccw
  arc A11 (-7.9799, 108.9908) -> (-47.4515, 102.3148) centre (-21.6467, 69.7703) ccw
  arc A12 (-47.4515, 102.3148) -> (-63.1417, 98.5922) centre (-49.1128, 74.3896) ccw
  arc A13 (-63.1417, 98.5922) -> (-59.3268, 82.3482) centre (-7.2967, 103.1374) ccw
  arc A14 (-59.3268, 82.3482) -> (-56.18, 60.807) centre (-22.274, 76.7606) ccw
  arc A15 (-56.18, 60.807) -> (-44.4039, 51.4337) centre (-38.8296, 70.521) ccw
  arc A16 (-44.4039, 51.4337) -> (-44.4564, 49.3124) centre (-36.8862, 50.1866) ccw
  line L8 (-44.4564, 49.3124) -> (-69.3262, 49.3124)
  arc A17 (-69.3262, 49.3124) -> (-74.3262, 44.3124) centre (-69.3262, 44.3124) ccw
  line L9 (-74.3262, 44.3124) -> (-74.3262, -60.6876)
  line L10 (-44.4564, 49.3124) -> (9.0437, 49.3124)
  circle A18 centre (-24.9939, 75.8846) radius 3.3209
  circle A19 centre (-0.1255, 80.7619) radius 3.1762
  arc A20 (-11.8952, 75.1826) -> (-8.388, 77.1204) centre (-10.3157, 76.4668) ccw
  arc A21 (-14.3886, 75.3993) -> (-12.7722, 75.8077) centre (-13.7004, 76.0782) ccw
  arc A22 (-10.9231, 75.8846) -> (-12.7722, 75.8077) centre (-11.8296, 75.4131) ccw
  circle A23 centre (-15.0573, 75.8846) radius 0.5367
  arc A24 (-15.594, 75.8846) -> (-11.8952, 75.1826) centre (-13.6982, 75.7781) ccw
  arc A25 (-14.5207, 75.8846) -> (-14.3886, 75.3993) centre (-13.9134, 75.7892) ccw
  circle A26 centre (-8.9506, 77) radius 0.5754
  arc A27 (-10.9231, 75.8846) -> (-9.4738, 76.7606) centre (-10.3666, 76.6007) ccw
  ellipse E0 centre (-33.2977, 71.1388) end of major axis (-29.0152, 72.1012) minor radius 3.3846
  ellipse E1 centre (7.9216, 78.9212) end of major axis (11.701, 78.9212) minor radius 3.3363
  arc A28 (-60.2045, 96.9027) -> (-55.7006, 84.7939) centre (-35.6058, 99.1602) ccw
  arc A29 (-48.2962, 99.6239) -> (-60.2045, 96.9027) centre (-49.7484, 78.563) ccw
  arc A30 (-48.2962, 99.6239) -> (-55.7006, 84.7939) centre (180.8193, -24.0343) ccw
  arc A31 (4.7759, 108.7394) -> (-5.3771, 107.2849) centre (2.3244, 89.6887) ccw
  arc A32 (5.6457, 98.2443) -> (4.7759, 108.7394) centre (-22.2939, 101.2123) ccw
  arc A33 (5.6457, 98.2443) -> (-5.3771, 107.2849) centre (-17.9987, 80.656) ccw
  arc A34 (-34.1977, 58.7929) -> (-40.7944, 55.6926) centre (-31.7992, 45.1212) ccw
  arc A35 (-29.9803, 50.1866) -> (-34.1977, 58.7929) centre (-46.6238, 47.3672) ccw
  arc A36 (-29.9803, 50.1866) -> (-32.4551, 49.3124) centre (-22.6105, 25.383) ccw
  line L11 (-43.378, 49.3124) -> (-32.4551, 49.3124)
  arc A37 (-28.7593, 52.3515) -> (-31.7992, 58.2512) centre (-30.1308, 55.3778) ccw
  arc A38 (-28.7593, 52.3515) -> (-31.7992, 58.2512) centre (-39.6355, 50.4803) ccw
  arc A39 (-28.0547, 49.3124) -> (-28.3148, 50.6217) centre (-30.1832, 49.57) ccw
  arc A40 (-28.3148, 50.6217) -> (-26.1924, 53.1861) centre (-29.2478, 53.5544) ccw
  arc A41 (-26.1924, 53.1861) -> (4.7759, 60.9485) centre (-21.929, 101.8324) ccw
  line L12 (-28.0547, 49.3124) -> (7.4717, 49.3124)
  arc A42 (11.2898, 58.1666) -> (7.1874, 61.3766) centre (8.8379, 59.2595) ccw
  arc A43 (4.6929, 59.7202) -> (9.194, 54.9482) centre (17.407, 67.2036) ccw
  arc A44 (4.6929, 59.7202) -> (7.1874, 61.3766) centre (-2.3382, 73.0155) ccw
  arc A45 (9.194, 54.9482) -> (11.2898, 58.1666) centre (1.5602, 62.2108) ccw
  arc A46 (6.1831, 49.3124) -> (9.8951, 53.7224) centre (-9.9172, 66.6317) ccw
  arc A47 (2.6622, 59.6434) -> (8.9309, 52.3515) centre (15.7837, 64.5832) ccw
  arc A48 (-40.7944, 55.6926) -> (-42.5331, 49.3124) centre (-36.497, 51.0944) ccw
  arc A49 (-55.5312, -38.35) -> (-54.5312, -39.35) centre (-54.5312, -38.35) ccw projected
  line L13 (-55.5312, -38.35) -> (-55.5312, 38.35) projected
  arc A50 (-54.5312, 39.35) -> (-55.5312, 38.35) centre (-54.5312, 38.35) ccw projected
  line L14 (-54.5312, 39.35) -> (59.7692, 39.35) projected
  arc A51 (59.7692, 39.35) -> (60.7692, 40.35) centre (59.7692, 40.35) ccw projected
  line L15 (60.7692, 40.35) -> (60.7692, 48.35) projected
  arc A52 (60.7692, 48.35) -> (59.7692, 49.35) centre (59.7692, 48.35) ccw projected
  line L16 (59.7692, 49.35) -> (9.0839, 49.35) projected
  arc A53 (9.0839, 49.35) -> (12.1204, 53.0639) centre (-3.3832, 62.6419) ccw projected
  arc A54 (12.1204, 53.0639) -> (11.1906, 54.2327) centre (-35.0005, 16.5336) ccw projected
  arc A55 (11.1906, 54.2327) -> (14.3248, 58.2512) centre (-10.3438, 74.2601) ccw projected
  arc A56 (14.3248, 58.2512) -> (11.1906, 63.387) centre (11.2567, 59.9031) ccw projected
  arc A57 (11.1906, 63.387) -> (11.701, 82.5854) centre (-0.1255, 73.2938) ccw projected
  arc A58 (11.701, 82.5854) -> (7.5139, 96.445) centre (-17.5403, 81.3137) ccw projected
  arc A59 (7.5139, 96.445) -> (6.1831, 110.8888) centre (-24.9939, 100.7331) ccw projected
  arc A60 (6.1831, 110.8888) -> (-7.9799, 108.9908) centre (1.8063, 89.7576) ccw projected
  arc A61 (-7.9799, 108.9908) -> (-47.4515, 102.3148) centre (-21.6467, 69.7703) ccw projected
  arc A62 (-47.4515, 102.3148) -> (-63.1417, 98.5922) centre (-49.1128, 74.3896) ccw projected
  arc A63 (-63.1417, 98.5922) -> (-59.3268, 82.3482) centre (-7.2967, 103.1374) ccw projected
  arc A64 (-59.3268, 82.3482) -> (-56.18, 60.807) centre (-22.274, 76.7606) ccw projected
  arc A65 (-56.18, 60.807) -> (-44.4039, 51.4337) centre (-38.8296, 70.521) ccw projected
  arc A66 (-44.4039, 51.4337) -> (-44.4606, 49.35) centre (-36.8862, 50.1866) ccw projected
  line L17 (-44.4606, 49.35) -> (-60.5312, 49.35) projected
  arc A67 (-60.5312, 49.35) -> (-65.5312, 44.35) centre (-60.5312, 44.35) ccw projected
  line L18 (-65.5312, 44.35) -> (-65.5312, -44.35) projected
  arc A68 (-65.5312, -44.35) -> (-60.5312, -49.35) centre (-60.5312, -44.35) ccw projected
  line L19 (-60.5312, -49.35) -> (64.5312, -49.35) projected
  arc A69 (64.5312, -49.35) -> (65.5312, -48.35) centre (64.5312, -48.35) ccw projected
  line L20 (65.5312, -48.35) -> (65.5312, -40.35) projected
  arc A70 (65.5312, -40.35) -> (64.5312, -39.35) centre (64.5312, -40.35) ccw projected
  line L21 (64.5312, -39.35) -> (-54.5312, -39.35) projected
  point P0 (0, 0)
  point P1 (0, 0)
  point P2 (4.147, 60.5446)
  dimension "d31" = 90
  constraints: 99 point on circle, 51 centre point, 18 end point, 6 point on line, 3 horizontal, 2 other
  measures "d31" distance of L2.end L0.start
extrude "Extrusion8" cut sketch "Sketch9" against normal blind 2 contours A48 A34 A35 A36 L10 | A39 A40 A41 A47 A46 L10 | A18 | A19 | A24 A23 A25 A21 A22 A27 A26 A20 | A26 | A23 A25 | E0 | E1 | A29 A30 A28 | A32 A33 A31 | A38 A37 | A45 A43 A44 A42 picked at (-15.2321, 75.8308)
body "Solid1"
